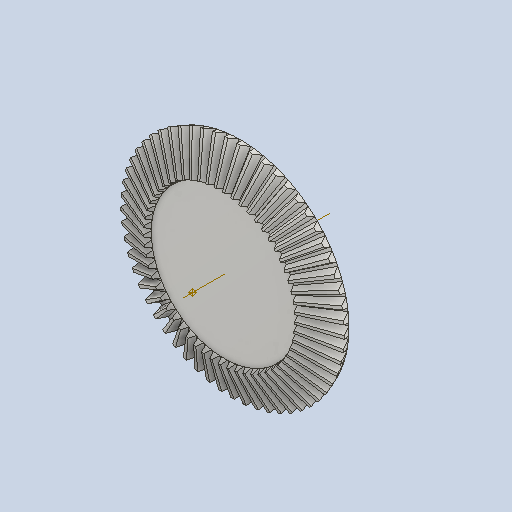
# Autodesk Inventor part: Bevel Gear2
Saved by Autodesk Inventor 2024 (Build 280153000, 153)
## iProperties
Created: 2024-03-20
Part Number: Bevel Gear2
Material: Steel, Mild
Document SubType Name: Modeling
Designer: mater
Categories: <?xml version="1.0" encoding="UTF-16"?> <MemberInstance><Categories><FamilyTemplate><FamilyTemplateParameter ValueType="xs:double" Id="1" ObjectReferenceKey="da_z" ObjectType="kUserParameterObject"/><FamilyTemplateParameter ValueType="xs:double" Id="2" ObjectReferenceKey="da_b" ObjectType="kUserParameterObject"/><FamilyTemplateParameter ValueType="xs:double" Id="3" ObjectReferenceKey="da_beta" ObjectType="kUserParameterObject"/><FamilyTemplateParameter ValueType="xs:double" Id="4" ObjectReferenceKey="da_dae" ObjectType="kUserParameterObject"/><FamilyTemplateParameter ValueType="xs:double" Id="5" ObjectReferenceKey="da_ve" ObjectType="kUserParameterObject"/><FamilyTemplateParameter ValueType="xs:double" Id="6" ObjectReferenceKey="da_omega" ObjectType="kUserParameterObject"/><FamilyTemplateParameter ValueType="xs:string" Id="7" ObjectReferenceKey="EAIAABAAAAAAHwAAAAAAAIAAAAAAAAAA" ObjectType="83914240" SubObjectId="SurfaceGeometry"/></FamilyTemplate><ParamToTemplateMap><ParamToTemplate CategoryParameter="//CategoryParameter[@InternalName='046C89C9-8512-4d59-83FE-43B91F4F132A']" TemplateParameter="1"/><ParamToTemplate CategoryParameter="//CategoryParameter[@InternalName='2552DF32-E462-4b46-AEBF-C6C7768E72AC']" TemplateParameter="2"/><ParamToTemplate CategoryParameter="//CategoryParameter[@InternalName='C9EE641D-15FC-4fae-A226-E94C4372FDD7']" TemplateParameter="3"/><ParamToTemplate><ParamToTemplate CategoryParameter="//CategoryParameter[@InternalName='00B6519A-459B-49c7-AD84-2E56D39A5744']" ConstantValue="-0.000000"/></ParamToTemplate><ParamToTemplate><ParamToTemplate CategoryParameter="//CategoryParameter[@InternalName='04B31F0E-C7A6-4894-AA32-9629BEFACF47']" ConstantValue="1.000000"/></ParamToTemplate><ParamToTemplate><ParamToTemplate CategoryParameter="//CategoryParameter[@InternalName='43CBEC2E-7847-49e7-A936-2F7889FCB2D9']" ConstantValue="0.200000"/></ParamToTemplate><ParamToTemplate><ParamToTemplate CategoryParameter="//CategoryParameter[@InternalName='B1EFC894-105D-4ebd-86BF-FA20ED196853']" ConstantValue="0.300000"/></ParamToTemplate><ParamToTemplate><ParamToTemplate CategoryParameter="//CategoryParameter[@InternalName='51175063-3D10-4879-93E8-6246FE8B403D']" ConstantValue="2061532430.657340"/></ParamToTemplate><ParamToTemplate><ParamToTemplate CategoryParameter="//CategoryParameter[@InternalName='A3A52E27-4454-46a9-B0BD-C932399B70AF']" ConstantValue="0.300000"/></ParamToTemplate><ParamToTemplate CategoryParameter="//CategoryParameter[@InternalName='2A200944-5A8C-41ca-B96E-8520D2E510F1']" TemplateParameter="4"/><ParamToTemplate><ParamToTemplate CategoryParameter="//CategoryParameter[@InternalName='1A637F62-92C8-44bc-B81F-10802510B579']" ConstantValue="9.895298"/></ParamToTemplate><ParamToTemplate CategoryParameter="//CategoryParameter[@InternalName='B52DD4BE-6863-48fb-BF58-89EF6F9EC65C']" TemplateParameter="5"/><ParamToTemplate><ParamToTemplate CategoryParameter="//CategoryParameter[@InternalName='3956BFF2-84D2-457d-93C2-9B0613DEBA67']" ConstantValue="1.811644"/></ParamToTemplate><ParamToTemplate CategoryParameter="//CategoryParameter[@InternalName='739CFA02-461B-4bf8-8049-181FCAD8B28F']" TemplateParameter="6"/><ParamToTemplate><ParamToTemplate CategoryParameter="//CategoryParameter[@InternalName='A27E999F-E2CE-4481-8A2A-EBF499C4C3C5']" ConstantValue="-0.000000"/></ParamToTemplate><ParamToTemplate><ParamToTemplate CategoryParameter="//CategoryParameter[@InternalName='9E1B4470-B2D3-4ff1-B813-535BB4CDF51A']" ConstantValue="3523220.976809"/></ParamToTemplate><ParamToTemplate><ParamToTemplate CategoryParameter="//CategoryParameter[@InternalName='F8452263-BFF6-458c-9FB1-07C4B99E95CD']" ConstantValue="11397033.805607"/></ParamToTemplate><ParamToTemplate><ParamToTemplate CategoryParameter="//CategoryParameter[@InternalName='3E3BB259-FD49-497f-8171-6EBC954A3479']" ConstantValue="2.000000"/></ParamToTemplate><ParamToTemplate CategoryParameter="//CategoryParameter[@InternalName='27C3BAF2-7550-4e4b-AE2C-0DB134B7D9B7']" TemplateParameter="7"/></ParamToTemplateMap><Category DisplayName="Gear" InternalName="DC85795E-93AB-48d5-8EEE-5A27447B64BD" Mnemonic="Gear"><CategoryParameter DisplayName="z" InternalName="046C89C9-8512-4d59-83FE-43B91F4F132A" Mnemonic="z"/><CategoryParameter DisplayName="b" InternalName="2552DF32-E462-4b46-AEBF-C6C7768E72AC" Mnemonic="b"/><CategoryParameter DisplayName="||b|" InternalName="C9EE641D-15FC-4fae-A226-E94C4372FDD7" Mnemonic="beta"/><CategoryParameter DisplayName="x" InternalName="00B6519A-459B-49c7-AD84-2E56D39A5744" Mnemonic="x"/><CategoryParameter DisplayName="a*" InternalName="04B31F0E-C7A6-4894-AA32-9629BEFACF47" Mnemonic="a"/><CategoryParameter DisplayName="c*" InternalName="43CBEC2E-7847-49e7-A936-2F7889FCB2D9" Mnemonic="c"/><CategoryParameter DisplayName="r|.f|*" InternalName="B1EFC894-105D-4ebd-86BF-FA20ED196853" Mnemonic="rf"/><CategoryParameter DisplayName="E" InternalName="51175063-3D10-4879-93E8-6246FE8B403D" Mnemonic="E"/><CategoryParameter DisplayName="||m|" InternalName="A3A52E27-4454-46a9-B0BD-C932399B70AF" Mnemonic="mi"/><Category DisplayName="BevelGear" InternalName="0C98F69A-0C2B-4791-B2FE-7691BB227E77" Mnemonic="BevelGear"><CategoryParameter DisplayName="d|.ae|" InternalName="2A200944-5A8C-41ca-B96E-8520D2E510F1" Mnemonic="dae"/><CategoryParameter DisplayName="d|.ai|" InternalName="1A637F62-92C8-44bc-B81F-10802510B579" Mnemonic="dai"/><CategoryParameter DisplayName="A|.e|" InternalName="B52DD4BE-6863-48fb-BF58-89EF6F9EC65C" Mnemonic="ve"/><CategoryParameter DisplayName="A|.i|" InternalName="3956BFF2-84D2-457d-93C2-9B0613DEBA67" Mnemonic="vi"/><CategoryParameter DisplayName="||S|" InternalName="739CFA02-461B-4bf8-8049-181FCAD8B28F" Mnemonic="omega"/><CategoryParameter DisplayName="x|.t|" InternalName="A27E999F-E2CE-4481-8A2A-EBF499C4C3C5" Mnemonic="xt"/><CategoryParameter DisplayName="||s||.Flim|" InternalName="9E1B4470-B2D3-4ff1-B813-535BB4CDF51A" Mnemonic="sFlim"/><CategoryParameter DisplayName="||s||.Hlim|" InternalName="F8452263-BFF6-458c-9FB1-07C4B99E95CD" Mnemonic="sHlim"/><CategoryParameter DisplayName="type" InternalName="3E3BB259-FD49-497f-8171-6EBC954A3479" Mnemonic="type"/><CategoryParameter DisplayName="PitchDiameter" InternalName="27C3BAF2-7550-4e4b-AE2C-0DB134B7D9B7" Mnemonic="IDS_PITCHDIAM"/></Category></Category></Categories></MemberInstance>
Mass: 60.9118 g
Surface Area: 34.3074 cm^2
Volume: 7.7496 cm^3
Density: 7.86 g/cm^3
Appearance: Steel
CustomPartVersion: 1
Author: mater
Autodesk Inventor part; units mm, degrees
ref_plane "Mesh Plane2" through (0, 0, 0) normal (0.9984815, 0.0550878, 0) x (0, 0, 1)
sketch "Teeth Body Sketch" plane through (0, 0, 0) normal (1, 0, 0) x (0, 1, 0)
  line L0 (0, 0) -> (71.2495, -32.0366) construction
  line L1 (71.2495, -32.0366) -> (73.3405, -26.8545)
  line L2 (73.3405, -26.8545) -> (0, 0) construction
  line L3 (72.39, -29.21) -> (0, 0) construction
  line L4 (48.0659, -21.6123) -> (49.4765, -18.1164)
  line L5 (71.2495, -32.0366) -> (48.0659, -21.6123)
  line L6 (73.3405, -26.8545) -> (49.4765, -18.1164)
  line L7 (0, -39.3868) -> (0, 6.5645) projected
  line L8 (0, -29.21) -> (73.3405, -29.21) construction
  dimension "d0" = 144.78
  dimension "d1" = 142.4989
  dimension "d2" = 146.6809
  dimension "d3" = 25.4
  dimension "d4" = 26.8545
  constraints: 16 end point, 4 point on line, 3 perpendicular, 2 collinear, 1 horizontal alignment, 1 vertical alignment
  measures "d0" diameter of L3.start L7
  measures "d1" diameter of L0.end L7
  measures "d2" diameter of L1.end L7
  measures "d3" distance between parallel lines of L1 L4
  measures "d4" vertical distance of L1.end L0.start
revolve "Teeth Body" add sketch "Teeth Body Sketch" angle 360 about axis through (0, 0, 0) along (0, 0, 1)
ref_plane "Tooth Plane" through (0, 72.39, -29.21) normal (0, -0.9273504, 0.374194) x (1, 0, 0)
sketch "Start Sketch" plane through (0, 72.39, -29.21) normal (0, -0.9273504, 0.374194) x (1, 0, 0)
  line L0 (0, -23.5051) -> (0, 10.6448) projected
  arc A0 (-0.7779, -3.7186) -> (-3.6689, 4.1824) centre (-65.0679, -22.764) ccw
  arc A1 (3.6689, 4.1824) -> (0.7779, -3.7186) centre (65.0679, -22.764) ccw
  line L1 (-0.7779, -3.7186) -> (0.7779, -3.7186)
  arc A2 (3.6689, 4.1824) -> (-3.6689, 4.1824) centre (0, -193.4558) ccw
  dimension "d7" = 67.0517
  dimension "d8" = 65.0679
  dimension "d9" = 170.6918
  dimension "d57" = 197.6722
  dimension "d58" = 189.7372
  constraints: 6 point on circle, 3 centre point, 3 symmetric about line, 2 end point, 1 coincident, 1 perpendicular, 1 other
  measures "d7" radius of A0
  measures "d8" horizontal distance of point (0, -193.456) A0.centre
  measures "d9" vertical distance of point (0, -193.456) A0.centre
  measures "d57" radius of A2
  measures "d58" distance from line of A2.centre L1
sketch "End Sketch" plane through (0, 48.5762, -19.6009) normal (0, -0.9273504, 0.374194) x (1, 0, 0)
  line L0 (0, -15.354) -> (0, 6.9534) projected
  arc A0 (-0.522, -2.4953) -> (-2.462, 2.8065) centre (-43.6628, -15.2754) ccw
  arc A1 (2.462, 2.8065) -> (0.522, -2.4953) centre (43.6628, -15.2754) ccw
  line L1 (-0.522, -2.4953) -> (0.522, -2.4953)
  arc A2 (2.462, 2.8065) -> (-2.462, 2.8065) centre (0, -129.8155) ccw
  dimension "d12" = 44.994
  dimension "d15" = 43.6628
  dimension "d16" = 114.5401
  dimension "d59" = 132.6449
  dimension "d60" = 127.3203
  constraints: 6 point on circle, 3 centre point, 3 symmetric about line, 2 end point, 1 coincident, 1 other
  measures "d12" radius of A0
  measures "d15" horizontal distance of A0.centre point (0, -129.816)
  measures "d16" vertical distance of A0.centre point (0, -129.816)
  measures "d59" radius of A2
  measures "d60" distance from line of A2.centre L1
loft "Loft" cut profiles "Start Sketch", "End Sketch"
pattern_circular "Circular Pattern" count 57 over 360 about axis through (0, 0, 0) along (0, 0, 1) of "Loft"
ref_plane "End Plane" through (0, 48.5762, -19.6009) normal (0, -0.9273504, 0.374194) x (1, 0, 0)
sketch3d "3D Sketch Right"
ref_plane "End Plane Right" through (-7.4609, 47.9998, -19.6009) normal (0.1424324, -0.916347, 0.374194) x (0.9881345, 0.1535907, 0)
sketch "End Sketch Right" plane through (-7.4609, 47.9998, -19.6009) normal (0.1424324, -0.916347, 0.374194) x (0.9881345, 0.1535907, 0)
  arc A0 (-0.522, -2.4953) -> (-2.462, 2.8065) centre (-43.6628, -15.2754) ccw
  line L0 (0, -157.5776) -> (0, 31.5287) projected
  arc A1 (2.462, 2.8065) -> (0.522, -2.4953) centre (43.6628, -15.2754) ccw
  line L1 (-0.522, -2.4953) -> (0.522, -2.4953)
  arc A2 (2.462, 2.8065) -> (-2.462, 2.8065) centre (0, -129.8155) ccw
  dimension "d70" = 43.6628
  dimension "d71" = 114.5401
  dimension "d72" = 44.994
  dimension "d73" = 127.3203
  dimension "d74" = 132.6449
  constraints: 6 point on circle, 3 centre point, 3 symmetric about line, 2 end point, 1 coincident, 1 perpendicular, 1 other
  measures "d70" horizontal distance of A2.centre A0.centre
  measures "d71" vertical distance of point (0, -129.816) A0.centre
  measures "d72" radius of A0
  measures "d73" distance from line of point (0, -129.816) L1
  measures "d74" radius of A2
feature "Loft Right" [suppressed]
pattern_circular "Circular Pattern Right" [suppressed]
sketch3d "3D Sketch Left"
ref_plane "End Plane Left" through (7.5604, 47.9998, -19.6791) normal (-0.1442138, -0.9155855, 0.375374) x (0.9878215, -0.1555917, 0)
sketch "End Sketch Left" plane through (7.5604, 47.9998, -19.6791) normal (-0.1442138, -0.9155855, 0.375374) x (0.9878215, -0.1555917, 0)
  line L0 (0, -158.5764) -> (0, 32.5966) projected
  arc A0 (-0.522, -2.4285) -> (-2.462, 2.8733) centre (-43.6628, -15.2087) ccw
  arc A1 (2.462, 2.8733) -> (0.522, -2.4285) centre (43.6628, -15.2087) ccw
  line L1 (-0.522, -2.4285) -> (0.522, -2.4285)
  ellipse E0 centre (0, -16.7916) end of major axis (49.4765, -16.7916) minor radius 18.5722 projected
  arc A2 (2.462, 2.8733) -> (-2.462, 2.8733) centre (0, -129.7488) ccw
  dimension "d56" = 18.5722
  dimension "d30" = 44.994
  dimension "d31" = 43.6628
  dimension "d32" = 114.5401
  dimension "d61" = 132.6449
  dimension "d62" = 127.3203
  constraints: 6 point on circle, 3 centre point, 3 symmetric about line, 2 end point, 1 coincident, 2 other
  measures "d30" radius of A0
  measures "d31" horizontal distance of point (0, -129.749) A0.centre
  measures "d32" vertical distance of A0.centre point (0, -129.749)
  measures "d61" radius of A2
  measures "d62" distance from line of point (0, -129.749) L1
feature "Loft Left" [suppressed]
pattern_circular "Circular Pattern Left" [suppressed]
sketch "Body Sketch" plane through (0, 0, 0) normal (1, 0, 0) x (0, 1, 0)
  line L0 (0, -35.0375) -> (0, -19.5308) projected
  line L1 (71.2495, -32.0366) -> (48.0659, -21.6123) projected
  line L2 (48.0659, -21.6123) -> (0, -21.6123)
  line L3 (71.2495, -32.0366) -> (0, -32.0366)
  constraints: 4 end point, 2 perpendicular, 2 point on line
revolve "Fix Body" add sketch "Body Sketch" angle 360 about axis through (0, 0, 0) along (0, 0, 1)
sketch "Sketch6" plane through (0, 0, 0) normal (1, 0, 0) x (0, 1, 0)
  line L0 (72.39, -29.21) -> (0, 0) projected
  line L1 (0, -37.7999) -> (0, 6.3) projected
surface revolve "Pitch Diameter" sketch "Sketch6" angle 360 about axis through (0, 0, 0) along (0, 0, 1) shown no curves L0
equation "\"d0\" = da_de"
equation "\"d1\" = da_dfe"
equation "\"d2\" = da_dae"
equation "\"d3\" = da_b"
equation "\"d4\" = da_ve"
equation "\"d7\" = fd_rr"
equation "\"d8\" = fd_x"
equation "\"d9\" = fd_y"
equation "\"d57\" = 0.5 * fd_dva + 0.3 * da_he"
equation "\"d58\" = 0.5 * fd_dva - 1.12 * da_he"
equation "\"da_teethtype\" = 0"
equation "\"da_b\" = 25.4"
equation "\"da_de\" = 144.78"
equation "\"da_dae\" = 146.68091"
equation "\"da_dfe\" = 142.49891"
equation "\"da_le\" = 78.06111"
equation "\"da_omega\" = 90deg"
equation "\"da_beta\" = 0"
equation "\"da_delta\" = 68.025492deg"
equation "\"da_alpha\" = 20deg"
equation "\"da_he\" = 5.588"
equation "\"da_ve\" = 26.85453"
equation "\"da_zv\" = 152.327388"
equation "\"fd_loft\" = da_b + 0.05 * da_he"
equation "\"fd_x\" = fd_x1 + fd_x2"
equation "\"fd_y\" = fd_y1 - fd_y2"
equation "\"fd_dd\" = fd_dva - 0.8 * da_he"
equation "\"da_dvw\" = 386.91157"
equation "\"d11\" = fd_loft"
equation "\"da_dm\" = 121.2253"
equation "\"da_x\" = 0"
equation "\"da_m\" = 2.54"
equation "\"d50\" = da_omega"
equation "\"fd_rr\" = 67.051721"
equation "\"fd_dva\" = 391.991567"
equation "\"fd_x1\" = 1.994876"
equation "\"fd_x2\" = 63.07299"
equation "\"fd_y1\" = 193.445498"
equation "\"fd_y2\" = 22.75371"
body "Solid1"
body "Srf1"
